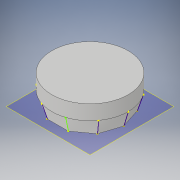
# Autodesk Inventor part: Probe P1.5
Saved by Autodesk Inventor 2019 (Build 230136000, 136)
## iProperties
Created: 2019-07-29
Part Number: Probe P1.5
Material: Generic
Document SubType Name: Modeling
Designer: azriel
Density: 1 g/cm^3
Appearance: Default
Author: azriel
Autodesk Inventor part; units mm, degrees
ref_plane "YZ Plane" through (0, 0, 0) normal (1, 0, 0) x (0, 1, 0)
ref_plane "XZ Plane" through (0, 0, 0) normal (0, 1, 0) x (-1, 0, 0)
ref_plane "XY Plane" through (0, 0, 0) normal (0, 0, 1) x (1, 0, 0)
sketch "Sketch1" plane through (0, 0, 0) normal (0, 1, 0) x (-1, 0, 0)
  circle A0 centre (0, 0) radius 13
  line L0 (-11.5, 0) -> (-9.3037, 6.7595) construction
  line L1 (-9.3037, 6.7595) -> (-3.5537, 10.9371) construction
  line L2 (-3.5537, 10.9371) -> (3.5537, 10.9371) construction
  line L3 (3.5537, 10.9371) -> (9.3037, 6.7595) construction
  line L4 (9.3037, 6.7595) -> (11.5, 0) construction
  line L5 (11.5, 0) -> (9.3037, -6.7595) construction
  line L6 (9.3037, -6.7595) -> (3.5537, -10.9371) construction
  line L7 (3.5537, -10.9371) -> (-3.5537, -10.9371) construction
  line L8 (-3.5537, -10.9371) -> (-9.3037, -6.7595) construction
  line L9 (-9.3037, -6.7595) -> (-11.5, 0) construction
  circle A1 centre (-6, 0) radius 3 construction
  circle A2 centre (6, 0) radius 3 construction
  line L10 (13, 0) -> (10.5172, -7.6412) construction
  line L11 (10.5172, -7.6412) -> (4.0172, -12.3637) construction
  line L12 (4.0172, -12.3637) -> (-4.0172, -12.3637) construction
  line L13 (-4.0172, -12.3637) -> (-10.5172, -7.6412) construction
  line L14 (-10.5172, -7.6412) -> (-13, 0) construction
  line L15 (-13, 0) -> (-10.5172, 7.6412) construction
  line L16 (-10.5172, 7.6412) -> (-4.0172, 12.3637) construction
  line L17 (-4.0172, 12.3637) -> (4.0172, 12.3637) construction
  line L18 (4.0172, 12.3637) -> (10.5172, 7.6412) construction
  line L19 (10.5172, 7.6412) -> (13, 0) construction
  dimension "d0" = 26
  dimension "d10" = 6
  dimension "d11" = 6
  constraints: 40 end point, 2 centre point, 2 coincident, 1 horizontal alignment, 23 other
  measures "d10" diameter of A1
  measures "d11" diameter of A2
ref_plane "Work Plane1" through (0, -5, 0) normal (0, -1, 0) x (1, 0, 0)
sketch "Sketch2" plane through (0, -5, 0) normal (0, -1, 0) x (1, 0, 0)
  circle A0 centre (0, 0) radius 13 construction
  line L0 (-9.3037, 6.7595) -> (-11.5, 0) projected
  line L1 (-11.5, 0) -> (-9.3037, 6.7595)
  line L2 (-9.3037, 6.7595) -> (-3.5537, 10.9371)
  line L3 (-3.5537, 10.9371) -> (3.5537, 10.9371)
  line L4 (3.5537, 10.9371) -> (9.3037, 6.7595)
  line L5 (9.3037, 6.7595) -> (11.5, 0)
  line L6 (11.5, 0) -> (9.3037, -6.7595)
  line L7 (9.3037, -6.7595) -> (3.5537, -10.9371)
  line L8 (3.5537, -10.9371) -> (-3.5537, -10.9371)
  line L9 (-3.5537, -10.9371) -> (-9.3037, -6.7595)
  line L10 (-9.3037, -6.7595) -> (-11.5, 0)
  constraints: 20 end point, 2 coincident, 1 centre point, 21 other
sketch3d "3D Sketch1"
loft "Loft1" add profiles "Sketch1", "Sketch2"
sketch "Sketch3" plane through (0, 0, 0) normal (0, 1, 0) x (1, 0, 0)
  circle A0 centre (0, 0) radius 13
  constraints: 1 centre point, 1 coincident
extrude "Extrusion3" add sketch "Sketch3" along normal blind 5
body "Solid2"
